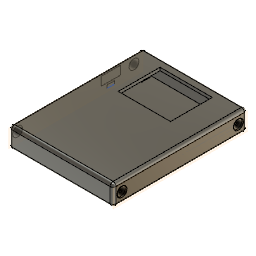
FirstAidCard_liurunkun (Autodesk Fusion 360 design; units mm, degrees)
Autodesk Fusion 360 part; units mm, degrees
sketch "Sketch1" plane through (0, 0, 0) normal (0, 0, 1) x (1, 0, 0) in component "Case"
  line L0 (-35, 45) -> (35, 45)
  line L1 (35, 45) -> (35, -45)
  line L2 (35, -45) -> (-35, -45)
  line L3 (-35, -45) -> (-35, 45)
  dimension "d1" = 90
  dimension "d2" = 45
  dimension "d3" = 35
  dimension "d6" = 70
  constraint horizontal L0
  constraint vertical L1
  constraint horizontal L2
  constraint vertical L3
  measures "d1" distance of L0.start L2.end
  measures "d2" vertical distance of origin L0.start
  measures "d3" horizontal distance of origin L0.start
  measures "d6" distance of L0.start L0.end
extrude "Extrude1" add sketch "Sketch1" along normal blind 12 makes body 1 in component "Case"
shell "Shell1" thickness 2 removed faces 1 at (-11.6667, -15, 12) on bodies 1 in component "Case"
sketch "Sketch3" plane through (-35, 0, 0) normal (-1, 0, 0) x (0, -1, 0) in component "Case"
  line L0 (-45, 0) -> (45, 0)
  line L1 (45, 0) -> (45, 12)
  line L2 (45, 12) -> (-45, 12)
  line L3 (-45, 12) -> (-45, 0)
  circle A0 centre (-39, 7) radius 3.25
  circle A1 centre (39, 7) radius 3.25
  line L4 (-30, 11) -> (-17, 11)
  line L5 (-17, 11) -> (-17, 5.2)
  line L6 (-17, 5.2) -> (-30, 5.2)
  line L7 (-30, 5.2) -> (-30, 11)
  line L8 (-26, 4) -> (-21, 4)
  line L9 (-21, 4) -> (-21, 2)
  line L10 (-21, 2) -> (-26, 2)
  line L11 (-26, 2) -> (-26, 4)
  dimension "d18" = 6.5
  dimension "d19" = 6
  dimension "d20" = 5
  dimension "d21" = 6.5
  dimension "d22" = 6
  dimension "d23" = 5
  dimension "d47" = 13
  dimension "d48" = 5.8
  dimension "d49" = 1
  dimension "d50" = 15
  dimension "d51" = 5
  dimension "d52" = 4
  dimension "d53" = 19
  constraint horizontal L4
  constraint vertical L5
  constraint horizontal L6
  constraint vertical L7
  constraint horizontal L8
  constraint vertical L9
  constraint horizontal L10
  constraint vertical L11
  measures "d18" diameter of A0
  measures "d19" horizontal distance of L2.end A0.centre
  measures "d20" vertical distance of L2.end A0.centre
  measures "d21" diameter of A1
  measures "d22" horizontal distance of L1.end A1.centre
  measures "d23" vertical distance of L1.end A1.centre
  measures "d47" distance of L4.start L4.end
  measures "d48" distance of L4.start L6.end
  measures "d49" vertical distance of L2.end L4.start
  measures "d50" horizontal distance of L2.end L4.start
  measures "d51" distance of L8.start L8.end
  measures "d52" vertical distance of L0.start L8.start
  measures "d53" horizontal distance of L0.start L8.start
extrude "Extrude5" cut sketch "Sketch3" against normal blind 4 contours L4 L5 L6 L7 | L8 L9 L10 L11 bodies 1 in component "Case"
hole "Hole2" at (-35, -39, 7) direction (1, 0, 0) diameter 2 depth 6 tip angle 118 bodies 1 in component "Case"
hole "Hole1" at (-35, 39, 7) direction (1, 0, 0) diameter 2 depth 6 tip angle 118 bodies 1 in component "Case"
extrude "Extrude3" cut sketch "Sketch3" against normal blind 1 contours A0 | A1 bodies 1 in component "Case"
sketch "Sketch4" plane through (35, 0, 0) normal (1, 0, 0) x (0, 1, 0) in component "Case"
  line L0 (-45, 0) -> (45, 0)
  line L1 (45, 0) -> (45, 12)
  line L2 (45, 12) -> (-45, 12)
  line L3 (-45, 12) -> (-45, 0)
  circle A0 centre (-39, 7) radius 3.25
  circle A1 centre (39, 7) radius 3.25
  dimension "d32" = 6.5
  dimension "d33" = 6
  dimension "d34" = 5
  dimension "d35" = 6.5
  dimension "d36" = 6
  dimension "d37" = 5
  measures "d32" diameter of A0
  measures "d33" horizontal distance of L2.end A0.centre
  measures "d34" vertical distance of L2.end A0.centre
  measures "d35" diameter of A1
  measures "d36" horizontal distance of L1.end A1.centre
  measures "d37" vertical distance of L1.end A1.centre
hole "Hole4" at (35, -39, 7) direction (-1, 0, 0) diameter 2 depth 6 tip angle 118 bodies 1 in component "Case"
hole "Hole3" at (35, 39, 7) direction (-1, 0, 0) diameter 2 depth 6 tip angle 118 bodies 1 in component "Case"
extrude "Extrude4" cut sketch "Sketch4" against normal blind 1 contours A0 | A1 bodies 1 in component "Case"
fillet "Fillet1" radius 2 8 edges at (-35, -45, 6) (0, -45, 0) (35, -45, 6) (35, 0, 0) (35, 45, 6) (0, 45, 0) (-35, 45, 6) (-35, 0, 0) on bodies 1 in component "Case"
sketch "Sketch1 (2)" plane through (0, 0, 12) normal (0, 0, 1) x (-1, 0, 0) in component "Top"
  line L0 (33, 43) -> (33, -43)
  line L1 (33, -43) -> (-33, -43)
  line L2 (-33, -43) -> (-33, 43)
  line L3 (-33, 43) -> (33, 43)
  arc A0 (35, 43) -> (33, 45) centre (33, 43) ccw
  line L4 (33, 45) -> (-33, 45)
  arc A1 (-33, 45) -> (-35, 43) centre (-33, 43) ccw
  line L5 (-35, 43) -> (-35, -43)
  arc A2 (-35, -43) -> (-33, -45) centre (-33, -43) ccw
  line L6 (-33, -45) -> (33, -45)
  arc A3 (33, -45) -> (35, -43) centre (33, -43) ccw
  line L7 (35, -43) -> (35, 43)
  line L8 (33, -21) -> (33, 43)
  line L9 (33, 43) -> (-33, 43)
  line L10 (-33, 43) -> (-33, -43)
  line L11 (-33, -43) -> (33, -43)
  line L12 (33, -43) -> (33, -26)
  line L13 (33, -26) -> (35, -26)
  line L14 (35, -26) -> (35, -21)
  line L15 (35, -21) -> (33, -21)
extrude "Extrude1'" add sketch "Sketch1 (2)" along normal blind 2 separate body makes body 2 in component "Top"
sketch "Sketch2" plane through (0, 0, 12) normal (0, 0, -1) x (1, 0, 0) in component "Top"
  line L0 (-35, 43) -> (-35, -43)
  arc A0 (-35, -43) -> (-33, -45) centre (-33, -43) ccw
  line L1 (-33, -45) -> (33, -45)
  arc A1 (33, -45) -> (35, -43) centre (33, -43) ccw
  line L2 (35, -43) -> (35, 43)
  arc A2 (35, 43) -> (33, 45) centre (33, 43) ccw
  line L3 (33, 45) -> (-33, 45)
  arc A3 (-33, 45) -> (-35, 43) centre (-33, 43) ccw
  line L4 (33, 42) -> (27, 42)
  line L5 (27, 42) -> (27, 36)
  line L6 (27, 36) -> (33, 36)
  line L7 (33, 36) -> (33, 42)
  line L8 (-33, 42) -> (-27, 42)
  line L9 (-27, 42) -> (-27, 36)
  line L10 (-27, 36) -> (-33, 36)
  line L11 (-33, 36) -> (-33, 42)
  line L12 (-33, -42) -> (-27, -42)
  line L13 (-27, -42) -> (-27, -36)
  line L14 (-27, -36) -> (-33, -36)
  line L15 (-33, -36) -> (-33, -42)
  line L16 (33, -36) -> (27, -36)
  line L17 (27, -36) -> (27, -42)
  line L18 (27, -42) -> (33, -42)
  line L19 (33, -42) -> (33, -36)
  dimension "d58" = 6
  dimension "d59" = 6
  dimension "d60" = 3
  dimension "d61" = 2
  dimension "d62" = 6
  dimension "d63" = 6
  dimension "d64" = 3
  dimension "d65" = 2
  dimension "d66" = 6
  dimension "d67" = 6
  dimension "d68" = 2
  dimension "d69" = 3
  dimension "d70" = 6
  dimension "d71" = 6
  dimension "d72" = 3
  dimension "d73" = 2
  constraint horizontal L4
  constraint vertical L5
  constraint horizontal L6
  constraint vertical L7
  constraint horizontal L8
  constraint vertical L9
  constraint horizontal L10
  constraint vertical L11
  constraint horizontal L12
  constraint vertical L13
  constraint horizontal L14
  constraint vertical L15
  constraint horizontal L16
  constraint vertical L17
  constraint horizontal L18
  constraint vertical L19
  measures "d58" distance of L4.start L4.end
  measures "d59" distance of L4.start L6.end
  measures "d60" vertical distance of A2.end L4.start
  measures "d61" horizontal distance of L2.end L4.start
  measures "d62" distance of L8.start L8.end
  measures "d63" distance of L8.start L10.end
  measures "d64" vertical distance of L3.end L8.start
  measures "d65" horizontal distance of L0.start L8.start
  measures "d66" distance of L12.start L12.end
  measures "d67" distance of L12.start L14.end
  measures "d68" horizontal distance of L0.end L12.start
  measures "d69" distance of A0.end L12.start
  measures "d70" distance of L16.start L16.end
  measures "d71" distance of L16.start L18.end
  measures "d72" vertical distance of L1.end L18.end
  measures "d73" horizontal distance of A1.end L18.end
extrude "Extrude2" add sketch "Sketch2" along normal blind 10 contours L4 L5 L6 L7 | L8 L9 L10 L11 | L12 L13 L14 L15 | L16 L17 L18 L19 bodies 2 in component "Top"
hole "Hole1'" at (33, 39, 7) direction (-1, 0, 0) diameter 2 depth 6 tip angle 118 bodies 2 in component "Top"
hole "Hole2'" at (33, -39, 7) direction (-1, 0, 0) diameter 2 depth 6 tip angle 118 bodies 2 in component "Top"
hole "Hole3'" at (-33, -39, 7) direction (1, 0, 0) diameter 2 depth 6 tip angle 118 bodies 2 in component "Top"
hole "Hole4'" at (-33, 39, 7) direction (1, 0, 0) diameter 2 depth 6 tip angle 118 bodies 2 in component "Top"
sketch "Sketch3 (2)" plane through (0, 0, 14) normal (0, 0, 1) x (-1, 0, 0) in component "Top"
  line L0 (35, -43) -> (35, 43)
  arc A0 (35, 43) -> (33, 45) centre (33, 43) ccw
  line L1 (33, 45) -> (-33, 45)
  arc A1 (-33, 45) -> (-35, 43) centre (-33, 43) ccw
  line L2 (-35, 43) -> (-35, -43)
  arc A2 (-35, -43) -> (-33, -45) centre (-33, -43) ccw
  line L3 (-33, -45) -> (33, -45)
  arc A3 (33, -45) -> (35, -43) centre (33, -43) ccw
  line L4 (17.5, -39) -> (-17.5, -39)
  line L5 (-17.5, -39) -> (-17.5, -11)
  line L6 (-17.5, -11) -> (17.5, -11)
  line L7 (17.5, -11) -> (17.5, -39)
  dimension "d88" = 35
  dimension "d89" = 28
  dimension "d90" = 17.5
  dimension "d91" = 6
  constraint horizontal L4
  constraint vertical L5
  constraint horizontal L6
  constraint vertical L7
  measures "d88" distance of L4.start L4.end
  measures "d89" distance of L4.start L6.end
  measures "d90" horizontal distance of origin L4.start
  measures "d91" vertical distance of L3.end L4.start
extrude "Extrude3'" cut sketch "Sketch3 (2)" against normal blind 4 contours L4 L5 L6 L7 bodies 2 in component "Top"
fillet "Fillet1'" radius 2 8 edges at (34.4142, 44.4142, 14) (0, 45, 14) (-34.4142, 44.4142, 14) (-35, 0, 14) (-34.4142, -44.4142, 14) (0, -45, 14) (34.4142, -44.4142, 14) (35, 0, 14) on bodies 2 in component "Top"
component "Top" placed x (1, 0, 0) y (0, 1, 0) z (0, 0, 1) at (0, 0, 0)
component "Case" placed x (1, 0, 0) y (0, 1, 0) z (0, 0, 1) at (0, 0, 0)
